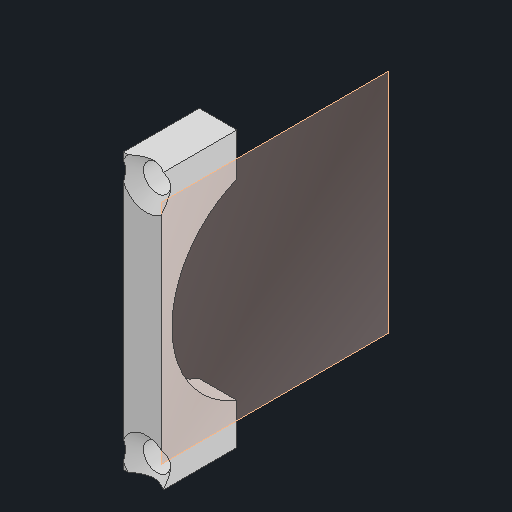
# Autodesk Inventor part: right_motor_ceil_2
Saved by Autodesk Inventor 2023 (Build 270158000, 158)
## iProperties
Created: 2024-04-14
Part Number: right_motor_ceil_2
Material: Generic
Document SubType Name: Modeling
Designer: szymo
Density: 1 g/cm^3
Appearance: Default
Author: szymo
Autodesk Inventor part; units mm, degrees
ref_plane "YZ Plane" through (0, 0, 0) normal (1, 0, 0) x (0, 1, 0)
ref_plane "XZ Plane" through (0, 0, 0) normal (0, 1, 0) x (-1, 0, 0)
ref_plane "Work Plane1" through (5, 13.3547, -3.0565) normal (1, 0, 0) x (0, -1, 0)
ref_plane "Work Plane2" through (0, -4.8088, -18.4315) normal (-1, 0, 0) x (0, 0, 1)
sketch "Sketch1" plane through (5, 13.3547, -3.0565) normal (1, 0, 0) x (0, -1, 0)
  arc A0 (6.1228, -3.0565) -> (-6.1228, -3.0565) centre (0, 0) ccw projected
  line L0 (6.1228, -3.0565) -> (18.1635, -3.0565) projected
  line L1 (18.1635, -3.0565) -> (18.1635, 15.375) projected
  line L2 (18.1635, 15.375) -> (-18.375, 15.375) projected
  line L3 (-18.375, 15.375) -> (-18.375, -3.0565) projected
  line L4 (-18.375, -3.0565) -> (-6.1228, -3.0565) projected
  circle A1 centre (8, 0) radius 1.0564 projected
  circle A2 centre (-8, 0) radius 1.0564 projected
  circle A3 centre (8, 0) radius 1.0564 projected
  circle A4 centre (-8, 0) radius 1.0564 projected
  circle A5 centre (0, 0) radius 5 projected
  circle A6 centre (0, 0) radius 13.7 projected
  line L5 (18.1635, 15.375) -> (18.1635, 1) projected
  line L6 (18.1635, 1) -> (13.6635, 1) projected
  arc A7 (13.6635, 1) -> (-13.6635, 1) centre (0, 0) ccw projected
  line L7 (-13.6635, 1) -> (-18.375, 1) projected
  line L8 (-18.375, 1) -> (-18.375, -15.125) projected
  line L9 (55.7975, -15.125) -> (-18.375, -15.125) projected
  line L10 (55.7975, -15.125) -> (55.7975, 5.375) projected
  line L11 (55.7975, 5.375) -> (48.7975, 5.375) projected
  line L12 (48.7975, 5.375) -> (48.7975, 15.375) projected
  line L13 (48.7975, 15.375) -> (18.1635, 15.375) projected
  line L14 (-18.375, -15.125) -> (18.1635, -15.125)
  line L15 (18.1635, -15.125) -> (18.1635, -5.0565)
  line L16 (18.1635, -5.0565) -> (-18.375, -5.0565)
  line L17 (-18.375, -5.0565) -> (-18.375, -15.125)
  circle A8 centre (0, 0) radius 9
  point P0 (13.3547, -3.0565)
  point P1 (7.4453, -5.0565)
  point P2 (-7.4453, -5.0565)
  point P3 (-18.375, -5.0565)
  point P4 (18.1635, -15.125)
  point P5 (12.7327, -5.0565)
  point P6 (-12.7327, -5.0565)
  dimension "d0" = 2
  dimension "d1" = 18
  constraints: 8 end point, 2 parallel, 1 centre point, 1 coincident, 1 collinear, 1 horizontal, 1 perpendicular
  measures "d0" distance between parallel lines of L16 L0
  measures "d1" diameter of A8
extrude "Extrusion1" add sketch "Sketch1" against normal up to surface (5 mm away) contours L16 L15 L9 L8 A6
sketch "Sketch2" plane through (5, -4.8088, 12.0685) normal (0, 0, 1) x (1, 0, 0)
  line L0 (-5, 4.8088) -> (0, 4.8088) projected
  line L1 (-5, 4.8088) -> (-5, 0) projected
  line L2 (-5, 0) -> (4.7, 0) projected
  line L3 (4.7, 12.0407) -> (4.7, 0) projected
  line L4 (0, 12.0407) -> (4.7, 12.0407) projected
  line L5 (0, 12.0407) -> (0, 4.8088) projected
  line L6 (-5, 36.5385) -> (4.7, 36.5385) projected
  line L7 (-5, 36.5385) -> (-5, 31.5181) projected
  line L8 (-5, 31.5181) -> (0, 31.5181) projected
  line L9 (0, 31.5181) -> (0, 24.2862) projected
  line L10 (0, 24.2862) -> (4.7, 24.2862) projected
  line L11 (4.7, 36.5385) -> (4.7, 24.2862) projected
  point P0 (-2, 2.2)
  point P1 (-2, 34.3385)
  dimension "d6" = 2.2
  dimension "d7" = 2.2
  dimension "d8" = 3
  dimension "d9" = 3
  measures "d6" distance from line of L2 point (-2, 2.2)
  measures "d7" distance from line of L6 point (-2, 34.338)
  measures "d8" distance from line of L7 point (-2, 34.338)
  measures "d9" distance from line of L1 point (-2, 2.2)
hole "Hole1" at (3, -2.6088, 12.0685) at (3, 29.5297, 12.0685) direction (0, 0, -1) diameter 3.6 end through all countersink diameter 6.5 countersink angle 90 clearance for "Countersunk Flat Head Screw ISO 2009/7046" size "M3" standard "ISO"
body "Solid1"
